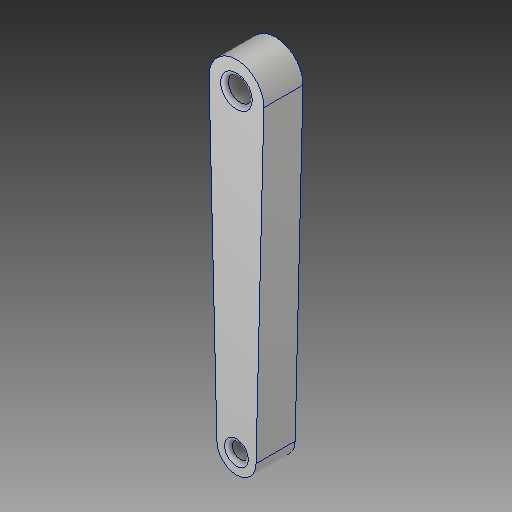
# Autodesk Inventor part: Upper Rocker Arm Spider Crab
Saved by Autodesk Inventor 2019 (Build 230136000, 136)
## iProperties
Created: 2019-08-25
Part Number: Upper Rocker Arm Spider Crab
Material: Aluminum 6061
Document SubType Name: Modeling
Designer: DIBYOJYOTI
Density: 2.7 g/cm^3
Appearance: Aluminum - Flat
Mass: 27.8773 g
Surface Area: 43.4018 cm^2
Volume: 10.3249 cm^3
Author: DIBYOJYOTI
Autodesk Inventor part; units mm, degrees
ref_plane "YZ Plane" through (0, 0, 0) normal (1, 0, 0) x (0, 1, 0)
ref_plane "XZ Plane" through (0, 0, 0) normal (0, 1, 0) x (-1, 0, 0)
ref_plane "XY Plane" through (0, 0, 0) normal (0, 0, 1) x (1, 0, 0)
sketch "Sketch1" plane through (0, 0, 0) normal (0, 0, 1) x (1, 0, 0)
  circle A0 centre (0, 0) radius 2.05
  circle A1 centre (0, 80) radius 3.05
  arc A2 (6.9978, 79.8249) -> (-6.9978, 79.8249) centre (0, 80) ccw
  arc A3 (-5, 0) -> (5, 0) centre (0, 0) ccw
  line L0 (-5, 0) -> (-6.9978, 79.8249)
  line L1 (5, 0) -> (6.9978, 79.8249)
  dimension "d0" = 4.1
  dimension "d3" = 6.1
  dimension "d5" = 80
  dimension "d12" = 14
  dimension "d13" = 10
  constraints: 4 centre point, 4 end point, 4 point on circle, 3 coincident, 2 tangent
  measures "d0" diameter of A0
  measures "d3" diameter of A1
  measures "d5" distance of point (0, 0) A1.centre
  measures "d12" diameter of A2
  measures "d13" diameter of A3
extrude "Extrusion3" add sketch "Sketch1" along normal blind 10
fillet "Fillet2" radius 1 4 edges at (-3.05, 80, 10) (-3.05, 80, 0) (-2.05, 0, 10) (-2.05, 0, 0)
body "Solid3"
